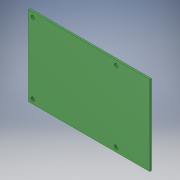
# Autodesk Inventor part: PiBoard
Saved by Autodesk Inventor 2018 (Build 220112000, 112)
## iProperties
Created: 2018-01-13
Part Number: PiBoard
Material: Thermoplastic Resin
Document SubType Name: Modeling
Designer: Kyle-HP
Density: 1.28 g/cm^3
Appearance: Smooth - Dark Forest Green
Author: Kyle-HP
Autodesk Inventor part; units mm, degrees
ref_plane "YZ Plane" through (0, 0, 0) normal (1, 0, 0) x (0, 1, 0)
ref_plane "XZ Plane" through (0, 0, 0) normal (0, 1, 0) x (-1, 0, 0)
ref_plane "XY Plane" through (0, 0, 0) normal (0, 0, 1) x (1, 0, 0)
sketch "Sketch1" plane through (0, 0, 0) normal (0, 0, 1) x (1, 0, 0)
  line L0 (0, 0) -> (85.09, 0)
  line L1 (85.09, 0) -> (85.09, -55.88)
  line L2 (85.09, -55.88) -> (0, -55.88)
  line L3 (0, -55.88) -> (0, 0)
  dimension "d0" = 85.09
  dimension "d1" = 55.88
  constraints: 8 end point, 2 parallel, 1 horizontal, 1 perpendicular
  measures "d0" distance of L0.start L0.end
  measures "d1" distance of L2.end L0.start
extrude "Extrusion1" add sketch "Sketch1" along normal blind 1.27
sketch "Sketch2" plane through (0, 0, 1.27) normal (0, 0, 1) x (1, 0, 0)
  circle A0 centre (3.175, -3.175) radius 1.27
  circle A1 centre (3.175, -52.705) radius 1.27
  circle A2 centre (61.595, -52.6948) radius 1.27
  circle A3 centre (61.595, -3.175) radius 1.27
  line L0 (85.09, 0) -> (0, 0) projected
  line L1 (0, 0) -> (0, -55.88) projected
  line L2 (0, -55.88) -> (85.09, -55.88) projected
  line L3 (85.09, -55.88) -> (85.09, 0) projected
  dimension "d4" = 2.54
  dimension "d5" = 2.54
  dimension "d6" = 2.54
  dimension "d7" = 2.54
  dimension "d8" = 3.175
  dimension "d9" = 3.175
  dimension "d10" = 3.175
  dimension "d11" = 3.175
  dimension "d12" = 3.1852
  dimension "d13" = 3.175
  dimension "d14" = 23.495
  dimension "d15" = 23.495
  constraints: 4 centre point
  measures "d4" diameter of A0
  measures "d5" diameter of A1
  measures "d6" diameter of A2
  measures "d7" diameter of A3
  measures "d8" distance from line of L0 A0.centre
  measures "d9" distance from line of L1 A0.centre
  measures "d10" distance from line of L1 A1.centre
  measures "d11" distance from line of L2 A1.centre
  measures "d12" distance from line of L2 A2.centre
  measures "d13" distance from line of L0 A3.centre
  measures "d14" distance from line of L3 A3.centre
  measures "d15" distance from line of L3 A2.centre
extrude "Extrusion2" cut sketch "Sketch2" against normal blind 1.27 contours A0 | A1 | A2 | A3
body "Solid1"
